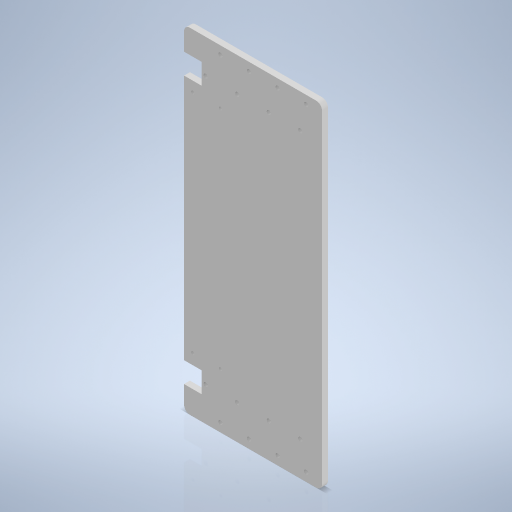
# Autodesk Inventor part: 1011
Saved by Autodesk Inventor 2024 (Build 280153000, 153)
## iProperties
Created: 2024-06-10
Part Number: 1011
Material: Generisch
Document SubType Name: Modeling
Designer: ffogue
Density: 1 g/cm^3
Appearance: Vorgabe
Author: ffogue
Autodesk Inventor part; units mm, degrees
ref_plane "YZ Plane" through (0, 0, 0) normal (1, 0, 0) x (0, 1, 0)
ref_plane "XZ Plane" through (0, 0, 0) normal (0, 1, 0) x (-1, 0, 0)
sketch "Skizze1" plane through (0, 0, 0) normal (0, 1, 0) x (-1, 0, 0)
  line L0 (-70, 170) -> (70, 170)
  line L1 (70, 170) -> (70, -170)
  line L2 (70, -170) -> (-70, -170)
  line L3 (-70, -170) -> (-70, 170)
  line L4 (-70, 170) -> (70, -170) construction
  line L5 (70, 170) -> (-70, -170) construction
  point P0 (0, 0)
  dimension "d0" = 340
  dimension "d1" = 140
  constraints: 12 end point, 2 midpoint, 2 parallel, 1 horizontal, 1 perpendicular
  measures "d0" distance between parallel lines of L2 L0
  measures "d1" distance between parallel lines of L3 L1
extrude "Extrusion1" add sketch "Skizze1" along normal blind 6
sketch "Skizze2" plane through (0, 6, 0) normal (0, 1, 0) x (1, 0, 0)
  line L0 (-70, 170) -> (-70, -170) projected
  line L1 (-70, -146) -> (-52, -146)
  line L2 (-52, -146) -> (-52, -125)
  line L3 (-52, -125) -> (-70, -125)
  line L4 (-70, 125) -> (-52, 125)
  line L5 (-52, 125) -> (-52, 146)
  line L6 (-52, 146) -> (-70, 146)
  line L7 (-70, -170) -> (70, -170) projected
  line L8 (70, 170) -> (-70, 170) projected
  point P0 (0, 0)
  dimension "d4" = 21
  dimension "d5" = 21
  dimension "d6" = 24
  dimension "d7" = 24
  dimension "d8" = 18
  constraints: 12 end point, 6 point on line, 3 perpendicular, 1 horizontal, 1 parallel
  measures "d4" distance of L4.end L5.end
  measures "d5" distance of L1.end L2.end
  measures "d6" distance between parallel lines of L7 L1
  measures "d7" distance between parallel lines of L8 L6
  measures "d8" distance between parallel lines of L0 L2
extrude "Extrusion2" cut sketch "Skizze2" against normal up to surface (6 mm away)
sketch "Skizze3" plane through (0, 6, 0) normal (0, 1, 0) x (1, 0, 0)
  line L0 (70, -170) -> (70, 170) projected
  line L1 (-52, -125) -> (-52, -146) projected
  point P0 (0, 0)
  point P1 (-48, -135.5)
  point P2 (-16, -135.5)
  point P3 (16, -135.5)
  point P4 (48, -135.5)
  point P5 (-52, -135.5)
  dimension "d11" = 22
  dimension "d12" = 32
  dimension "d13" = 32
  dimension "d14" = 32
  constraints: 4 horizontal alignment, 1 midpoint
  measures "d11" distance from line of L0 point (48, -135.5)
  measures "d12" distance of point (16, -135.5) point (48, -135.5)
  measures "d13" distance of point (16, -135.5) point (-16, -135.5)
  measures "d14" distance of point (-48, -135.5) point (-16, -135.5)
hole "Bohrung1" at (-48, 6, 135.5) at (-16, 6, 135.5) at (16, 6, 135.5) at (48, 6, 135.5) direction (0, -1, 0) diameter 4.134 depth 6 thread size "M5x0.8" class "6H" standard "ISO Metric profile"
fillet "Rundung1" radius 6 4 edges at (-70, 3, 170) (70, 3, 170) (70, 3, -170) (-70, 3, -170)
sketch "Skizze4" plane through (0, 6, 0) normal (0, 1, 0) x (1, 0, 0)
  circle A0 centre (48, -135.5) radius 2.067 projected
  line L0 (70, -164) -> (70, 164) projected
  point P0 (0, 0)
  point P1 (54, -161.5)
  point P2 (25, -161.5)
  point P3 (-4, -161.5)
  point P4 (-33, -161.5)
  dimension "d23" = 26
  dimension "d24" = 16
  dimension "d25" = 29
  dimension "d26" = 29
  dimension "d27" = 29
  constraints: 3 horizontal alignment
  measures "d23" vertical distance of A0.centre point (54, -161.5)
  measures "d24" distance from line of L0 point (54, -161.5)
  measures "d25" distance of point (25, -161.5) point (54, -161.5)
  measures "d26" distance of point (-4, -161.5) point (25, -161.5)
  measures "d27" distance of point (-33, -161.5) point (-4, -161.5)
hole "Bohrung2" at (54, 6, 161.5) at (25, 6, 161.5) at (-4, 6, 161.5) at (-33, 6, 161.5) direction (0, -1, 0) diameter 4.134 depth 6 thread size "M5x0.8" class "6H" standard "ISO Metric profile"
ref_plane "Arbeitsebene1" through (0, 0, 0) normal (0, 0, 1) x (1, 0, 0)
mirror "Spiegeln1" about plane through (0, 0, 0) normal (0, 0, 1) of "Bohrung2", "Bohrung1"
sketch "Skizze5" plane through (0, 6, 0) normal (0, 1, 0) x (1, 0, 0)
  line L0 (-70, -125) -> (-52, -125) projected
  point P0 (0, 0)
  point P1 (-61, -114.5)
  point P2 (-61, 114.5)
  point P3 (-61, -125)
  dimension "d36" = 114.5
  dimension "d37" = 114.5
  constraints: 2 vertical alignment, 1 midpoint
  measures "d36" vertical distance of point (-61, 114.5) point (0, 0)
  measures "d37" vertical distance of point (0, 0) point (-61, -114.5)
hole "Bohrung3" at (-61, 6, 114.5) at (-61, 6, -114.5) direction (0, -1, 0) diameter 3.242 depth 6 thread size "M4x0.7" class "6H" standard "ISO Metric profile"
sketch "Skizze6" plane through (0, 6, 0) normal (0, 1, 0) x (1, 0, 0)
  line L0 (-52, -125) -> (-52, -146) projected
  point P0 (0, 0)
  point P1 (-33, -114.5)
  point P2 (-33, 114.5)
  dimension "d45" = 19
  dimension "d46" = 114.5
  dimension "d47" = 114.5
  constraints: 1 vertical alignment
  measures "d45" distance from line of point (-33, -114.5) L0
  measures "d46" vertical distance of point (0, 0) point (-33, -114.5)
  measures "d47" vertical distance of point (0, 0) point (-33, 114.5)
hole "Bohrung4" at (-33, 6, 114.5) at (-33, 6, -114.5) direction (0, -1, 0) diameter 3.242 depth 6 thread size "M4x0.7" class "6H" standard "ISO Metric profile"
equation "\"d26\" = d25"
equation "\"d27\" = d25"
equation "\"d37\" = d36"
